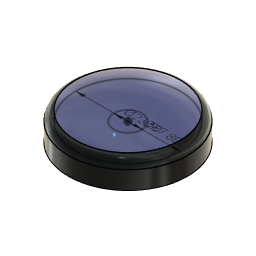
pjdcontrollerv27(no slider) (Autodesk Fusion 360 archive; units mm, degrees)
design "pjdbutton"
Autodesk Fusion 360 part; units mm, degrees
note: some values were not read from the file. Chosen so that the rebuilt part matches the saved one: that a step has no effect; which bodies a step acts on.
sketch "Sketch1" plane through (0, 0, 0) normal (0, 0, 1) x (1, 0, 0)
  circle A0 centre (0, 0) radius 50
  circle A1 centre (0, 0) radius 45
  dimension "d1" = 100
  dimension "d2" = 90
  constraint coincident A0.centre A1.centre
  measures "d1" diameter of A0
  measures "d2" diameter of A1
extrude "Extrude1" add sketch "Sketch1" along normal blind 15 makes body 1
ref_plane "WorkPlane1" through (0, 0, 15) normal (0, 0, 1) x (1, 0, 0)
sketch "Sketch2" plane through (0, 0, 15) normal (0, 0, 1) x (1, 0, 0)
  circle A0 centre (0, 0) radius 49.875
  circle A1 centre (0, 0) radius 43.9
  dimension "d6" = 99.75
  dimension "d7" = 87.8
  constraint coincident A0.centre A1.centre
  measures "d6" diameter of A0
  measures "d7" diameter of A1
extrude "Extrude2" add sketch "Sketch2" along normal blind 8 separate body contours A0 | A1 makes body 2
sketch "Sketch3" plane through (0, 0, 23) normal (0, 0, 1) x (-1, 0, 0)
  circle A0 centre (0, 0) radius 49.875
  circle A1 centre (0, 0) radius 43.9
  dimension "d10" = 87.8
  constraint coincident A0.centre A1.centre
  measures "d10" diameter of A1
extrude "Extrude3" add sketch "Sketch3" along normal blind 20.3 contours A1 bodies 2
fillet "Fillet1" radius 8 1 edges at (-46.4998, -18.0356, 23) on bodies 2
extrude "Extrude4" cut 1 faces at (7.3167, -8.3109, 43.3) along direction (0, 0, -1) blind 20.3 on bodies 2 bodies 2
extrude "Extrude5" add 1 faces at (9.4066, 4.1682, 23) along direction (0, 0, 1) blind 0.3 on bodies 2 bodies 2
sketch "Sketch4" plane through (0, 0, 0) normal (0, 1, 0) x (1, 0, 0)
  arc A0 (0, -35) -> (43.9, -23.3) centre (-2.6114, 63.0075) ccw
  line L0 (0, -35) -> (0, -23.3)
  line L1 (0, -23.3) -> (43.9, -23.3)
  constraint vertical L0
  constraint perpendicular L0 L1
revolve "Revolve1" add sketch "Sketch4" angle 360 about axis through (0, 0, 0) along (0, 0, -1) separate body makes body 3
sketch "Sketch5" plane through (0, 0, 15) normal (0, 0, -1) x (1, 0, 0)
  circle A0 centre (0, 0) radius 49.875
  circle A1 centre (0, 0) radius 43.9
  circle A2 centre (0, 0) radius 11.75
  dimension "d21" = 87.8
  dimension "d22" = 23.5
  constraint coincident A0.centre A1.centre
  constraint concentric A1 A2
  measures "d21" diameter of A1
  measures "d22" diameter of A2
extrude "Extrude6" add sketch "Sketch5" along normal blind 14 contours A1 bodies 1 2 3
extrude "Extrude7" add 1 faces at (-2.9694, 1.8719, 15) along direction (0, 0, -1) blind 15 on bodies 2 bodies 1 3 2
imported_body "Base Feature1" makes body 5 in component "91280A827"
move_body "Move1" bodies 5 to x (0, 0, -1) y (0, 1, 0) z (1, 0, 0) at (0, 0, 0) in component "91280A827"
move_body "Move2" bodies 5 to x (1, 0, 0) y (0, 1, 0) z (0, 0, 1) at (0, 0, 22.5) in component "91280A827"
move_body "Move3" bodies 5 to x (1, 0, 0) y (0, 1, 0) z (0, 0, 1) at (0, 0, -31) in component "91280A827"
combine "Combine1" [no effect]
copy_body "CutPasteBodies1" bodies 1 removing the originals makes body 6 in component "Component"
copy_body "CutPasteBodies1'" bodies 6 removing the originals makes body 7 in component "91280A827"
copy_body "CutPasteBodies2" bodies 3 removing the originals makes body 8 in component "Component"
extrude "Extrude8" add 1 faces at (-2.9694, 1.8719, 0) along direction (0, 0, -1) blind 20 on bodies 2 bodies 2
sketch "Sketch7" plane through (0, 0, 0) normal (0, 1, 0) x (1, 0, 0)
  line L0 (-11.75, 0) -> (-11.75, 0.5)
  line L1 (-11.75, 0) -> (-11.25, 0)
  line L2 (-11.25, 0) -> (-11.75, 0.5)
  line L3 (-11.75, 0.5) -> (-11.75, 1)
  line L4 (-11.75, 1) -> (-11.25, 1)
  line L5 (-11.25, 1) -> (-11.75, 0.5)
  dimension "d33" = 0.5
  dimension "d34" = 0.5
  constraint vertical L0
  constraint perpendicular L0 L1
  constraint perpendicular L1 L3
  constraint perpendicular L3 L4
  measures "d33" distance of L0.start L1.end
  measures "d34" distance of L0.end L3.end
extrude "Extrude9" cut 1 faces at (-2.9694, 1.8719, -20) along direction (0, 0, 1) blind 6 on bodies 2 bodies 2
thread "Thread1" "ISO Metric profile 24.0 M24x2 6g" major diameter 23.822 minor diameter 21.529 pitch 2 angle 60 modelled right hand crest width 0.2818 on face at (11.7354, 0.5857, -9) crest through (11.911, 0, -14.5) on bodies 2
component "91280A827" placed x (1, 0, 0) y (0, 1, 0) z (0, 0, 1) at (0, 0, 0)
component "Component" placed x (1, 0, 0) y (0, 1, 0) z (0, 0, 1) at (0, 0, 0)
